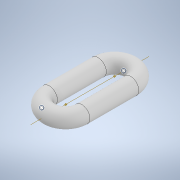
# Autodesk Inventor part: chainLink2
Saved by Autodesk Inventor 2020.3 (Build 243373000, 373)
## iProperties
Created: 2021-03-03
Part Number: chainLink2
Material: Generic
Document SubType Name: Modeling
Designer: con_c_000
Density: 1 g/cm^3
Appearance: Default
Author: con_c_000
Autodesk Inventor part; units mm, degrees
ref_plane "XZ Plane" through (0, 0, 0) normal (0, 1, 0) x (-1, 0, 0)
sketch "Sketch1" plane through (0, 0, 0) normal (0, 1, 0) x (-1, 0, 0)
  arc A0 (12.7, -9.7335) -> (0, -9.7335) centre (6.35, -9.7335) ccw
  arc A1 (0, -28.7835) -> (12.7, -28.7835) centre (6.35, -28.7835) ccw
  line L0 (12.7, -9.7335) -> (12.7, -28.7835)
  line L1 (0, -28.7835) -> (0, -9.7335)
  point P0 (0, 0)
  dimension "d0" = 12.7
  dimension "d1" = 12.7
  dimension "d2" = 19.05
  constraints: 4 end point, 4 point on circle, 3 tangent, 2 centre point, 1 vertical
  measures "d0" diameter of A0
  measures "d1" diameter of A1
  measures "d2" distance of A0.centre A1.centre
ref_plane "Work Plane1" through (0, 0, -19.05) normal (0, 0, 1) x (1, 0, 0)
sketch "Sketch2" plane through (0, 0, -19.05) normal (0, 0, 1) x (1, 0, 0)
  circle A0 centre (-12.7, 0) radius 3.175
  point P0 (0, 0)
  dimension "d4" = 6.35
  constraints: 1 centre point, 1 coincident
  measures "d4" diameter of A0
sweep "Sweep1" add profiles "Sketch2" path "Sketch1"
ref_plane "Work Plane2" through (-6.35, 0, -9.7335) normal (1, 0, 0) x (0, 0, -1)
body "Solid1"
